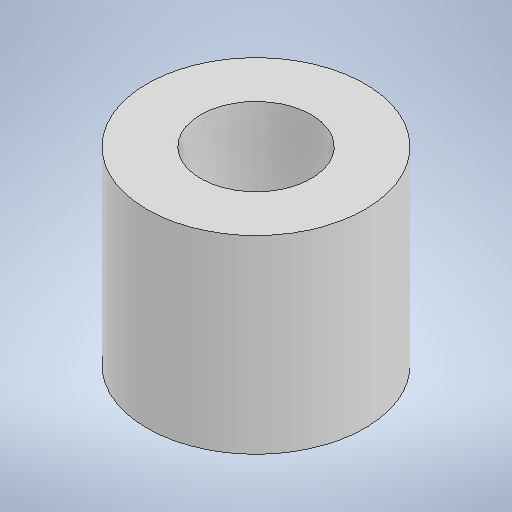
# Autodesk Inventor part: Standoff_Test
Saved by Autodesk Inventor 2025.1 (Build 291241020, 241B)
## iProperties
Created: 2024-11-21
Part Number: Standoff_Test
Material: Generic
Document SubType Name: Modeling
Designer: AtuStem
Density: 1 g/cm^3
Appearance: Default
Author: AtuStem
Autodesk Inventor part; units mm, degrees
ref_plane "YZ Plane" through (0, 0, 0) normal (1, 0, 0) x (0, 1, 0)
ref_plane "XZ Plane" through (0, 0, 0) normal (0, 1, 0) x (-1, 0, 0)
ref_plane "XY Plane" through (0, 0, 0) normal (0, 0, 1) x (1, 0, 0)
sketch "Sketch1" plane through (0, 0, 0) normal (0, 1, 0) x (-1, 0, 0)
  circle A0 centre (-2.9869, -30.5893) radius 3.7084
  circle A1 centre (-2.9869, 32.9107) radius 3.7084
  arc A2 (6.5381, 22.7507) -> (6.4048, 23.6608) centre (3.3631, 22.7507) ccw
  line L0 (4.1614, 34.4035) -> (6.4048, 23.6608)
  arc A3 (4.1614, 34.4035) -> (-10.1345, 34.407) centre (-2.9869, 32.9107) ccw
  line L1 (-12.3991, 23.5895) -> (-10.1345, 34.407)
  arc A4 (-12.3991, 23.5895) -> (-12.5119, 22.7507) centre (-9.3369, 22.7507) ccw
  line L2 (-12.5119, -21.6993) -> (-12.5119, 22.7507)
  arc A5 (-12.5119, -21.6993) -> (-12.3453, -22.7142) centre (-9.3369, -21.6993) ccw
  line L3 (-10.0947, -32.2643) -> (-12.3453, -22.7142)
  arc A6 (-10.0947, -32.2643) -> (4.1209, -32.2643) centre (-2.9869, -30.5893) ccw
  line L4 (6.3715, -22.7142) -> (4.1209, -32.2643)
  arc A7 (6.3715, -22.7142) -> (6.5381, -21.6993) centre (3.3631, -21.6993) ccw
  line L5 (6.5381, 22.7507) -> (6.5381, -21.6993)
  circle A8 centre (-2.9869, 32.9107) radius 7.3025
  point P0 (0, 0)
  point P1 (-2.9869, 7.5107)
  point P2 (-10.1345, 34.407)
  constraints: 12 end point, 12 point on circle, 9 centre point, 1 coincident
extrude "Extrusion1" add sketch "Sketch1" along normal blind 12.7 contours A8 A3
body "Solid1"
